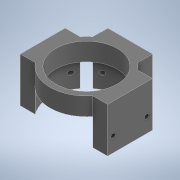
# Autodesk Inventor part: Battery and PI holder
Saved by Autodesk Inventor 2022 (Build 260153000, 153)
## iProperties
Created: 2023-01-18
Part Number: Battery and PI holder
Material: Generic
Document SubType Name: Modeling
Designer: ASUS
Density: 1 g/cm^3
Appearance: Gray
Author: ASUS
Autodesk Inventor part; units mm, degrees
ref_plane "YZ Plane" through (0, 0, 0) normal (1, 0, 0) x (0, 1, 0)
ref_plane "XZ Plane" through (0, 0, 0) normal (0, 1, 0) x (-1, 0, 0)
sketch "Sketch1" plane through (0, 0, 0) normal (0, 1, 0) x (-1, 0, 0)
  circle A0 centre (0, 0) radius 13.75
  circle A1 centre (0, 0) radius 16.25
  dimension "d0" = 27.5
  dimension "d5" = 32.5
  constraints: 2 centre point, 2 coincident
  measures "d0" diameter of A0
  measures "d5" diameter of A1
sketch "Sketch2" plane through (0, 0, 0) normal (0, 1, 0) x (-1, 0, 0)
  line L0 (21.5, 21.5) -> (-21.5, 21.5)
  line L1 (-21.5, 21.5) -> (-21.5, -21.5)
  line L2 (-21.5, -21.5) -> (21.5, -21.5)
  line L3 (21.5, -21.5) -> (21.5, 21.5)
  point P0 (0, 0)
  dimension "d1" = 43
  dimension "d2" = 43
  dimension "d3" = 21.5
  dimension "d4" = 21.5
  constraints: 8 end point, 2 parallel, 1 horizontal, 1 perpendicular
  measures "d1" distance of L2.end L0.start
  measures "d2" distance of L0.start L0.end
  measures "d3" distance from line of point (0, 0) L3
  measures "d4" distance from line of point (0, 0) L0
extrude "Extrusion1" add sketch "Sketch1" along normal blind 8
sketch "Sketch3" plane through (0, 8, 0) normal (0, 1, 0) x (1, 0, 0)
  line L0 (-17.7413, 16.25) -> (19.579, 16.25) construction
  line L1 (16.25, -18.4481) -> (16.25, 20.2858) construction
  line L2 (-16.25, -20.7099) -> (-16.25, 21.9822) construction
  line L3 (-16.5, 16.25) -> (16.5, 16.25) construction
  line L4 (16.5, 16.25) -> (16.5, 31.25) construction
  line L5 (16.5, 31.25) -> (-16.5, 31.25) construction
  line L6 (-16.5, 31.25) -> (-16.5, 16.25) construction
  circle A0 centre (0, 0) radius 16.25 projected
  line L7 (-16.25, -16.5) -> (-31.25, -16.5) construction
  line L8 (-31.25, -16.5) -> (-31.25, 16.5) construction
  line L9 (-31.25, 16.5) -> (-16.25, 16.5) construction
  line L10 (-16.25, 16.5) -> (-16.25, -16.5) construction
  line L11 (16.25, -16.5) -> (31.25, -16.5) construction
  line L12 (31.25, -16.5) -> (31.25, 16.5) construction
  line L13 (31.25, 16.5) -> (16.25, 16.5) construction
  line L14 (16.25, 16.5) -> (16.25, -16.5) construction
  line L15 (-16.5, -16.5) -> (16.25, -16.5)
  line L16 (16.5, 16.5) -> (16.5, 16.25)
  line L17 (-10, 12.8087) -> (-10, 16.5)
  line L18 (10, 12.8087) -> (10, 16.5)
  line L19 (16.5, 16.5) -> (-10, 16.5)
  line L20 (-16.25, 16.5) -> (-16.5, 16.5)
  line L21 (-16.5, 16.5) -> (-16.5, 16.25)
  line L22 (-16.5, 10) -> (-16.5, -10)
  line L23 (16.4416, -10) -> (16.4416, 10)
  circle A1 centre (0, 0) radius 16.25
  line L24 (-16.5, 10) -> (-12.8087, 10)
  line L25 (12.8087, 10) -> (16.4416, 10)
  line L26 (16.4416, -10) -> (12.8087, -10)
  line L27 (-12.8087, -10) -> (-16.5, -10)
  dimension "d8" = 33
  dimension "d9" = 15
  dimension "d10" = 16.5
  dimension "d11" = 15
  dimension "d12" = 16.5
  dimension "d13" = 33
  dimension "d14" = 16.5
  dimension "d15" = 15
  dimension "d16" = 33
  dimension "d20" = 10
  dimension "d21" = 10
  constraints: 56 end point, 16 perpendicular, 10 point on line, 6 parallel, 6 point on circle, 4 horizontal, 3 tangent, 3 vertical, 1 centre point, 1 coincident
  measures "d8" distance of L4.end L5.end
  measures "d9" distance of L5.end L3.start
  measures "d10" distance from line of L6 point (0, 0)
  measures "d11" distance of L7.start L7.end
  measures "d12" distance from line of point (0, 0) L7
  measures "d13" distance between parallel lines of L9 L7
  measures "d14" distance from line of point (0, 0) L11
  measures "d15" distance of L11.start L11.end
  measures "d16" distance of L11.end L12.end
  measures "d20" distance from line of point (0, 0) L17
  measures "d21" distance from line of point (0, 0) L18
extrude "Extrusion2" add sketch "Sketch3" against normal blind 20 contours A0 L25 L23 L26 | A0 L17 L19 L18 | L27 L22 L24 A0
sketch "Sketch4" plane through (16.4416, 8, 10) normal (1, 0, 0) x (0, 0, -1)
  line L0 (20, -20) -> (0, -20) projected
  line L1 (-3.75, 0) -> (23.75, 0) projected
  line L2 (-6.5, -20) -> (26.5, -20)
  line L3 (26.5, -20) -> (26.5, 0)
  line L4 (26.5, 0) -> (-6.5, 0)
  line L5 (-6.5, 0) -> (-6.5, -20)
  line L6 (10, 0) -> (10, -20) construction
  line L7 (2.5, 0) -> (2.5, -20) construction
  line L8 (17.5, 0) -> (17.5, -20) construction
  line L9 (-6.5, -13.5) -> (26.5, -13.5) construction
  line L10 (22.8087, -8) -> (20, -8) projected
  circle A0 centre (2.5, -13.5) radius 1
  circle A1 centre (17.5, -13.5) radius 1
  point P0 (10, -8)
  dimension "d26" = 33
  dimension "d27" = 20
  dimension "d28" = 16.5
  dimension "d29" = 7.5
  dimension "d30" = 7.5
  dimension "d31" = 5.5
  dimension "d32" = 2
  dimension "d33" = 2
  constraints: 16 end point, 11 point on line, 3 perpendicular, 2 centre point, 2 horizontal, 2 midpoint, 2 parallel
  measures "d26" distance of L2.start L2.end
  measures "d27" distance of L2.end L3.end
  measures "d28" distance from line of L3 point (10, -8)
  measures "d29" distance between parallel lines of L7 L6
  measures "d30" distance between parallel lines of L6 L8
  measures "d31" distance between parallel lines of L10 L9
  measures "d32" diameter of A0
  measures "d33" diameter of A1
extrude "Extrusion3" cut sketch "Sketch4" against normal through all contours A0 | A1
sketch "Sketch5" plane through (10, 8, -16.5) normal (0, 0, -1) x (-1, 0, 0)
  line L0 (-10.5226, -13.5) -> (32.3111, -13.5) construction
  line L1 (0, -8) -> (-2.8087, -8) projected
  circle A0 centre (2.5, -13.5) radius 1
  circle A1 centre (17.5, -13.5) radius 1
  point P0 (10, -8)
  dimension "d36" = 5.5
  dimension "d37" = 2
  dimension "d38" = 2
  dimension "d39" = 7.5
  dimension "d40" = 7.5
  constraints: 2 centre point, 2 end point, 2 point on line, 1 horizontal
  measures "d36" distance between parallel lines of L1 L0
  measures "d37" diameter of A0
  measures "d38" diameter of A1
  measures "d39" horizontal distance of point (10, -8) A0.centre
  measures "d40" horizontal distance of point (10, -8) A1.centre
extrude "Extrusion4" cut sketch "Sketch5" against normal through all
ref_plane "Work Plane1" through (0, 0, 16.25) normal (0, 0, 1) x (1, 0, 0)
sketch "Sketch9" plane through (16.4416, 8, 10) normal (1, 0, 0) x (0, 0, -1)
  line L0 (0, 0) -> (-6.25, 0) projected
  line L1 (20, -20) -> (0, -20) projected
  line L2 (0, 0) -> (20, 0)
  line L3 (20, 0) -> (20, -20)
  line L4 (20, -20) -> (0, -20)
  line L5 (0, -20) -> (0, 0)
  circle A0 centre (2.5, -13.5) radius 1 projected
  circle A1 centre (2.5, -13.5) radius 1
  circle A2 centre (17.5, -13.5) radius 1 projected
  circle A3 centre (17.5, -13.5) radius 1
  point P0 (10, -8)
  constraints: 8 end point, 2 centre point, 2 coincident, 2 parallel, 1 horizontal, 1 perpendicular
extrude "Extrusion7" add sketch "Sketch9" along normal blind 3
sketch "Sketch10" plane through (10, 8, -16.5) normal (0, 0, -1) x (-1, 0, 0)
  line L0 (-3.75, 0) -> (23.75, 0) projected
  line L1 (0, -8) -> (0, -20) projected
  line L2 (19.9113, 0) -> (0, 0)
  line L3 (0, 0) -> (0, -20)
  line L4 (0, -20) -> (19.9113, -20)
  line L5 (19.9113, -20) -> (19.9113, 0)
  circle A0 centre (17.5, -13.5) radius 1 projected
  circle A1 centre (17.5, -13.5) radius 1
  circle A2 centre (2.5, -13.5) radius 1 projected
  circle A3 centre (2.5, -13.5) radius 1
  point P0 (10, -8)
  constraints: 8 end point, 2 centre point, 2 coincident, 2 parallel, 1 horizontal, 1 perpendicular, 1 point on line
extrude "Extrusion8" add sketch "Sketch10" along normal blind 3
sketch "Sketch11" plane through (-16.5, 8, -10) normal (-1, 0, 0) x (0, 0, 1)
  line L0 (0, 0) -> (-2.8087, 0) projected
  line L1 (20, -20) -> (0, -20) projected
  line L2 (0, 0) -> (20, 0)
  line L3 (20, 0) -> (20, -20)
  line L4 (20, -20) -> (0, -20)
  line L5 (0, -20) -> (0, 0)
  circle A0 centre (17.5, -13.5) radius 1 projected
  circle A1 centre (17.5, -13.5) radius 1
  circle A2 centre (2.5, -13.5) radius 1 projected
  circle A3 centre (2.5, -13.5) radius 1
  point P0 (10, -8)
  constraints: 8 end point, 2 centre point, 2 coincident, 2 parallel, 1 horizontal, 1 perpendicular
extrude "Extrusion9" add sketch "Sketch11" along normal blind 3
sketch "Sketch6" plane through (0, 0, 16.25) normal (0, 0, 1) x (1, 0, 0)
  line L0 (10, 8) -> (-10, 8) projected
  line L1 (-10.5, 8) -> (10.5, 8)
  line L2 (10.5, 8) -> (10.5, -23)
  line L3 (10.5, -23) -> (-10.5, -23)
  line L4 (-10.5, -23) -> (-10.5, 8)
  circle A0 centre (-5.7, -21) radius 1
  circle A1 centre (5.7, -21) radius 1
  point P0 (0, 0)
  dimension "d44" = 21
  dimension "d45" = 10.5
  dimension "d46" = 31
  dimension "d47" = 2
  dimension "d48" = 2
  dimension "d49" = 4.8
  dimension "d50" = 4.8
  dimension "d51" = 2
  dimension "d52" = 2
  constraints: 8 end point, 2 centre point, 2 parallel, 1 horizontal, 1 perpendicular, 1 point on line
  measures "d44" distance of L2.end L3.end
  measures "d45" distance from line of point (0, 0) L4
  measures "d46" distance of L3.end L1.start
  measures "d47" diameter of A0
  measures "d48" diameter of A1
  measures "d49" distance from line of L4 A0.centre
  measures "d50" distance from line of L2 A1.centre
  measures "d51" distance from line of L3 A1.centre
  measures "d52" distance from line of L3 A0.centre
sketch "Sketch7" plane through (16.4416, 8, 10) normal (1, 0, 0) x (0, 0, -1)
  line L0 (0, -8) -> (0, -20) projected
  line L1 (20, -8) -> (20, 0) projected
  line L2 (0, -20) -> (20, -20)
  line L3 (20, -20) -> (20, 0)
  line L4 (20, 0) -> (0, 0)
  line L5 (0, 0) -> (0, -20)
  circle A0 centre (2.5, -13.5) radius 1 projected
  circle A1 centre (2.5, -13.5) radius 1
  circle A2 centre (17.5, -13.5) radius 1 projected
  circle A3 centre (17.5, -13.5) radius 1
  point P0 (10, -8)
  constraints: 8 end point, 2 centre point, 2 coincident, 2 parallel, 1 horizontal, 1 perpendicular
body "Solid1"
